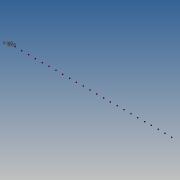
# Autodesk Inventor part: Part1
Saved by Autodesk Inventor 2020 (Build 240168000, 168)
## iProperties
Created: 2019-09-24
Part Number: Part1
Material: Generic
Document SubType Name: Modeling
Designer: a.komeijani
Density: 1 g/cm^3
Appearance: Default
Author: a.komeijani
Autodesk Inventor part; units mm, degrees
ref_plane "YZ Plane" through (0, 0, 0) normal (1, 0, 0) x (0, 1, 0)
ref_plane "XZ Plane" through (0, 0, 0) normal (0, 1, 0) x (-1, 0, 0)
ref_plane "XY Plane" through (0, 0, 0) normal (0, 0, 1) x (1, 0, 0)
sketch "Sketch1" plane through (0, 0, 0) normal (1, 0, 0) x (0, 1, 0)
  line L0 (-71.4801, 300) -> (29928.5199, 300)
  line L1 (29928.5199, 300) -> (29928.5199, 0)
  line L2 (29928.5199, 0) -> (-71.4801, 0)
  line L3 (-71.4801, 0) -> (-71.4801, 300)
  point P0 (0, 0)
  dimension "d0" = 30000
  dimension "d1" = 300
  constraints: 8 end point, 2 parallel, 1 horizontal, 1 perpendicular
  measures "d0" distance of L1.end L2.end
  measures "d1" distance of L2.end L0.start
extrude "Extrusion1" add sketch "Sketch1" along normal blind 50000
sketch "Sketch6" plane through (0, -71.4801, 300) normal (0, 0, 1) x (1, 0, 0)
  line L0 (0, 30000) -> (0, 0) projected
  circle A0 centre (0, 0) radius 2.5
  line L1 (3.2758, -2.2394) -> (5.0975, -2.2394)
  circle A1 centre (2000000, 0) radius 2.5
  circle A2 centre (4000000, 0) radius 2.5
  circle A3 centre (6000000, 0) radius 2.5
  circle A4 centre (8000000, 0) radius 2.5
  circle A5 centre (10000000, 0) radius 2.5
  circle A6 centre (12000000, 0) radius 2.5
  circle A7 centre (14000000, 0) radius 2.5
  circle A8 centre (16000000, 0) radius 2.5
  circle A9 centre (18000000, 0) radius 2.5
  circle A10 centre (20000000, 0) radius 2.5
  circle A11 centre (22000000, 0) radius 2.5
  circle A12 centre (24000000, 0) radius 2.5
  circle A13 centre (26000000, 0) radius 2.5
  circle A14 centre (28000000, 0) radius 2.5
  circle A15 centre (30000000, 0) radius 2.5
  circle A16 centre (32000000, 0) radius 2.5
  circle A17 centre (34000000, 0) radius 2.5
  circle A18 centre (36000000, 0) radius 2.5
  circle A19 centre (38000000, 0) radius 2.5
  circle A20 centre (40000000, 0) radius 2.5
  circle A21 centre (42000000, 0) radius 2.5
  circle A22 centre (44000000, 0) radius 2.5
  circle A23 centre (46000000, 0) radius 2.5
  circle A24 centre (48000000, 0) radius 2.5
  dimension "d21" = 5
  dimension "d24" = 2000000
  constraints: 25 centre point, 2 end point, 2 horizontal, 48 other
  measures "d21" diameter of A0
  measures "d24" distance of L0.end A1.centre
sketch "Sketch7" plane through (0, 0, 0) normal (-1, 0, 0) x (0, 0, 1)
  line L0 (300, 29928.5199) -> (300, -71.4801) projected
  point P0 (0, 0)
  point P1 (300, 29928.52)
body "Solid1"
